Autodesk Fusion 360 part; units mm, degrees
(part 3 of 6)
sketch "mv_std" plane through (-9.843, 0, 81.8196) normal (0, 1, 0) x (1, 0, 0)
  line L0 (174.293, 88.8196) -> (174.293, 74.8196)
  line L1 (40.943, 88.8196) -> (40.943, 74.8196)
  line L2 (131.143, 74.8196) -> (131.143, 88.8196)
  line L3 (112.093, 74.8196) -> (112.093, 88.8196)
  line L4 (35.893, 88.8196) -> (21.893, 88.8196)
  line L5 (98.093, 88.8196) -> (98.093, 74.8196)
  line L6 (2.843, 74.8196) -> (16.843, 74.8196)
  line L7 (174.293, 74.8196) -> (188.293, 74.8196)
  line L8 (2.843, 88.8196) -> (2.843, 74.8196)
  line L9 (21.893, 88.8196) -> (21.893, 74.8196)
  line L10 (150.193, 74.8196) -> (150.193, 88.8196)
  line L11 (16.843, 88.8196) -> (2.843, 88.8196)
  line L12 (59.993, 88.8196) -> (59.993, 74.8196)
  line L13 (131.143, 88.8196) -> (117.143, 88.8196)
  line L14 (98.093, 74.8196) -> (112.093, 74.8196)
  line L15 (21.893, 74.8196) -> (35.893, 74.8196)
  line L16 (35.893, 74.8196) -> (35.893, 88.8196)
  line L17 (188.293, 88.8196) -> (174.293, 88.8196)
  line L18 (59.993, 74.8196) -> (73.993, 74.8196)
  line L19 (188.293, 74.8196) -> (188.293, 88.8196)
  line L20 (16.843, 74.8196) -> (16.843, 88.8196)
  line L21 (54.943, 74.8196) -> (54.943, 88.8196)
  line L22 (73.993, 74.8196) -> (73.993, 88.8196)
  line L23 (73.993, 88.8196) -> (59.993, 88.8196)
  line L24 (40.943, 74.8196) -> (54.943, 74.8196)
  line L25 (117.143, 74.8196) -> (131.143, 74.8196)
  line L26 (54.943, 88.8196) -> (40.943, 88.8196)
  line L27 (155.243, 88.8196) -> (155.243, 74.8196)
  line L28 (136.193, 74.8196) -> (150.193, 74.8196)
  line L29 (112.093, 88.8196) -> (98.093, 88.8196)
  line L30 (79.043, 88.8196) -> (79.043, 74.8196)
  line L31 (150.193, 88.8196) -> (136.193, 88.8196)
  line L32 (93.043, 74.8196) -> (93.043, 88.8196)
  line L33 (169.243, 74.8196) -> (169.243, 88.8196)
  line L34 (93.043, 88.8196) -> (79.043, 88.8196)
  line L35 (193.343, 88.8196) -> (193.343, 74.8196)
  line L36 (40.6555, 55.7696) -> (40.6555, 69.7696)
  line L37 (79.043, 74.8196) -> (93.043, 74.8196)
  line L38 (19.2242, 55.7696) -> (19.2242, 69.7696)
  line L39 (117.143, 88.8196) -> (117.143, 74.8196)
  line L40 (26.6555, 55.7696) -> (40.6555, 55.7696)
  line L41 (26.6555, 69.7696) -> (26.6555, 55.7696)
  line L42 (207.343, 74.8196) -> (207.343, 88.8196)
  line L43 (155.243, 74.8196) -> (169.243, 74.8196)
  line L44 (219.5367, 88.8196) -> (219.5367, 74.8196)
  line L45 (207.343, 88.8196) -> (193.343, 88.8196)
  line L46 (45.7055, 55.7696) -> (59.7055, 55.7696)
  line L47 (233.5367, 88.8196) -> (219.5367, 88.8196)
  line L48 (19.2242, 69.7696) -> (5.2242, 69.7696)
  line L49 (59.7055, 69.7696) -> (45.7055, 69.7696)
  line L50 (59.7055, 55.7696) -> (59.7055, 69.7696)
  line L51 (136.193, 88.8196) -> (136.193, 74.8196)
  line L52 (219.5367, 74.8196) -> (233.5367, 74.8196)
  line L53 (5.2242, 55.7696) -> (19.2242, 55.7696)
  line L54 (5.2242, 69.7696) -> (5.2242, 55.7696)
  line L55 (193.343, 74.8196) -> (207.343, 74.8196)
  line L56 (233.5367, 74.8196) -> (233.5367, 88.8196)
  line L57 (40.6555, 69.7696) -> (26.6555, 69.7696)
  line L58 (169.243, 88.8196) -> (155.243, 88.8196)
  line L59 (160.0055, 69.7696) -> (160.0055, 55.7696)
  line L60 (9.9867, 50.7196) -> (9.9867, 36.7196)
  line L61 (97.8055, 55.7696) -> (97.8055, 69.7696)
  line L62 (78.7555, 55.7696) -> (78.7555, 69.7696)
  line L63 (135.9055, 55.7696) -> (135.9055, 69.7696)
  line L64 (235.918, 69.7696) -> (221.918, 69.7696)
  line L65 (45.7055, 69.7696) -> (45.7055, 55.7696)
  line L66 (36.1805, 36.7196) -> (50.1805, 36.7196)
  line L67 (50.1805, 36.7196) -> (50.1805, 50.7196)
  line L68 (107.3305, 36.7196) -> (107.3305, 50.7196)
  line L69 (140.9555, 55.7696) -> (154.9555, 55.7696)
  line L70 (107.3305, 50.7196) -> (93.3305, 50.7196)
  line L71 (126.3805, 36.7196) -> (126.3805, 50.7196)
  line L72 (36.1805, 50.7196) -> (36.1805, 36.7196)
  line L73 (198.1055, 55.7696) -> (212.1055, 55.7696)
  line L74 (64.7555, 55.7696) -> (78.7555, 55.7696)
  line L75 (78.7555, 69.7696) -> (64.7555, 69.7696)
  line L76 (121.9055, 55.7696) -> (135.9055, 55.7696)
  line L77 (9.9867, 36.7196) -> (23.9867, 36.7196)
  line L78 (145.4305, 36.7196) -> (145.4305, 50.7196)
  line L79 (116.8555, 69.7696) -> (102.8555, 69.7696)
  line L80 (164.4805, 50.7196) -> (150.4805, 50.7196)
  line L81 (112.3805, 36.7196) -> (126.3805, 36.7196)
  line L82 (112.3805, 50.7196) -> (112.3805, 36.7196)
  line L83 (131.4305, 36.7196) -> (145.4305, 36.7196)
  line L84 (93.3305, 50.7196) -> (93.3305, 36.7196)
  line L85 (179.0555, 55.7696) -> (193.0555, 55.7696)
  line L86 (164.4805, 36.7196) -> (164.4805, 50.7196)
  line L87 (102.8555, 69.7696) -> (102.8555, 55.7696)
  line L88 (23.9867, 50.7196) -> (9.9867, 50.7196)
  line L89 (74.2805, 50.7196) -> (74.2805, 36.7196)
  line L90 (121.9055, 69.7696) -> (121.9055, 55.7696)
  line L91 (140.9555, 69.7696) -> (140.9555, 55.7696)
  line L92 (126.3805, 50.7196) -> (112.3805, 50.7196)
  line L93 (145.4305, 50.7196) -> (131.4305, 50.7196)
  line L94 (174.0055, 55.7696) -> (174.0055, 69.7696)
  line L95 (50.1805, 50.7196) -> (36.1805, 50.7196)
  line L96 (150.4805, 50.7196) -> (150.4805, 36.7196)
  line L97 (83.8055, 55.7696) -> (97.8055, 55.7696)
  line L98 (97.8055, 69.7696) -> (83.8055, 69.7696)
  line L99 (83.8055, 69.7696) -> (83.8055, 55.7696)
  line L100 (193.0555, 69.7696) -> (179.0555, 69.7696)
  line L101 (235.918, 55.7696) -> (235.918, 69.7696)
  line L102 (174.0055, 69.7696) -> (160.0055, 69.7696)
  line L103 (64.7555, 69.7696) -> (64.7555, 55.7696)
  line L104 (150.4805, 36.7196) -> (164.4805, 36.7196)
  line L105 (74.2805, 36.7196) -> (88.2805, 36.7196)
  line L106 (212.1055, 69.7696) -> (198.1055, 69.7696)
  line L107 (131.4305, 50.7196) -> (131.4305, 36.7196)
  line L108 (154.9555, 55.7696) -> (154.9555, 69.7696)
  line L109 (179.0555, 69.7696) -> (179.0555, 55.7696)
  line L110 (212.1055, 55.7696) -> (212.1055, 69.7696)
  line L111 (154.9555, 69.7696) -> (140.9555, 69.7696)
  line L112 (116.8555, 55.7696) -> (116.8555, 69.7696)
  line L113 (193.0555, 55.7696) -> (193.0555, 69.7696)
  line L114 (31.418, 17.6696) -> (45.418, 17.6696)
  line L115 (57.6117, 31.6696) -> (57.6117, 17.6696)
  line L116 (169.5305, 50.7196) -> (169.5305, 36.7196)
  line L117 (153.8685, 17.6696) -> (153.8685, 32.6696)
  line L118 (69.2305, 36.7196) -> (69.2305, 50.7196)
  line L119 (233.5367, 31.6696) -> (219.5367, 31.6696)
  line L120 (82.5112, 17.6696) -> (89.5112, 17.6696)
  line L121 (221.918, 69.7696) -> (221.918, 55.7696)
  line L122 (57.6117, 17.6696) -> (71.6117, 17.6696)
  line L123 (131.4305, 17.6696) -> (145.4305, 17.6696)
  line L124 (240.6805, 36.7196) -> (240.6805, 50.7196)
  line L125 (188.5805, 31.6696) -> (188.5805, 17.6696)
  line L126 (145.4305, 31.6696) -> (131.4305, 31.6696)
  line L127 (183.5305, 36.7196) -> (183.5305, 50.7196)
  line L128 (221.918, 55.7696) -> (235.918, 55.7696)
  line L129 (207.6305, 36.7196) -> (221.6305, 36.7196)
  line L130 (19.2242, 31.6696) -> (5.2242, 31.6696)
  line L131 (202.5805, 36.7196) -> (202.5805, 50.7196)
  line L132 (71.6117, 31.6696) -> (57.6117, 31.6696)
  line L133 (219.5367, 17.6696) -> (233.5367, 17.6696)
  line L134 (89.5112, 17.6696) -> (89.5112, 32.6696)
  line L135 (226.6805, 50.7196) -> (226.6805, 36.7196)
  line L136 (55.2305, 50.7196) -> (55.2305, 36.7196)
  line L137 (93.3305, 36.7196) -> (107.3305, 36.7196)
  line L138 (122.9925, 17.6696) -> (129.9925, 17.6696)
  line L139 (198.1055, 69.7696) -> (198.1055, 55.7696)
  line L140 (135.9055, 69.7696) -> (121.9055, 69.7696)
  line L141 (113.3872, 32.6696) -> (106.3872, 32.6696)
  line L142 (129.9925, 17.6696) -> (129.9925, 32.6696)
  line L143 (207.6305, 50.7196) -> (207.6305, 36.7196)
  line L144 (5.2242, 31.6696) -> (5.2242, 17.6696)
  line L145 (188.5805, 50.7196) -> (188.5805, 36.7196)
  line L146 (90.9492, 17.6696) -> (104.9492, 17.6696)
  line L147 (162.3867, 17.6696) -> (176.3867, 17.6696)
  line L148 (202.5805, 50.7196) -> (188.5805, 50.7196)
  line L149 (162.3867, 31.6696) -> (162.3867, 17.6696)
  line L150 (183.5305, 50.7196) -> (169.5305, 50.7196)
  line L151 (19.2242, 17.6696) -> (19.2242, 31.6696)
  line L152 (90.9492, 31.6696) -> (90.9492, 17.6696)
  line L153 (176.3867, 17.6696) -> (176.3867, 31.6696)
  line L154 (82.5112, 32.6696) -> (82.5112, 17.6696)
  line L155 (88.2805, 36.7196) -> (88.2805, 50.7196)
  line L156 (160.0055, 55.7696) -> (174.0055, 55.7696)
  line L157 (221.6305, 36.7196) -> (221.6305, 50.7196)
  line L158 (129.9925, 32.6696) -> (122.9925, 32.6696)
  line L159 (71.6117, 17.6696) -> (71.6117, 31.6696)
  line L160 (233.5367, 17.6696) -> (233.5367, 31.6696)
  line L161 (102.8555, 55.7696) -> (116.8555, 55.7696)
  line L162 (188.5805, 36.7196) -> (202.5805, 36.7196)
  line L163 (202.5805, 17.6696) -> (202.5805, 31.6696)
  line L164 (113.3872, 17.6696) -> (113.3872, 32.6696)
  line L165 (219.5367, 31.6696) -> (219.5367, 17.6696)
  line L166 (45.418, 17.6696) -> (45.418, 31.6696)
  line L167 (55.2305, 36.7196) -> (69.2305, 36.7196)
  line L168 (88.2805, 50.7196) -> (74.2805, 50.7196)
  line L169 (176.3867, 31.6696) -> (162.3867, 31.6696)
  line L170 (146.8685, 32.6696) -> (146.8685, 17.6696)
  line L171 (23.9867, 36.7196) -> (23.9867, 50.7196)
  line L172 (240.6805, 50.7196) -> (226.6805, 50.7196)
  line L173 (221.6305, 50.7196) -> (207.6305, 50.7196)
  line L174 (106.3872, 32.6696) -> (106.3872, 17.6696)
  line L175 (226.6805, 36.7196) -> (240.6805, 36.7196)
  line L176 (45.418, 31.6696) -> (31.418, 31.6696)
  line L177 (69.2305, 50.7196) -> (55.2305, 50.7196)
  line L178 (169.5305, 36.7196) -> (183.5305, 36.7196)
  line L179 (106.3872, 17.6696) -> (113.3872, 17.6696)
  line L180 (188.5805, 17.6696) -> (202.5805, 17.6696)
  line L181 (31.418, 31.6696) -> (31.418, 17.6696)
  line L182 (104.9492, 17.6696) -> (104.9492, 31.6696)
  line L183 (202.5805, 31.6696) -> (188.5805, 31.6696)
  line L184 (104.9492, 31.6696) -> (90.9492, 31.6696)
  line L185 (89.5112, 32.6696) -> (82.5112, 32.6696)
  line L186 (5.2242, 17.6696) -> (19.2242, 17.6696)
  line L187 (122.9925, 32.6696) -> (122.9925, 17.6696)
  line L188 (146.8685, 17.6696) -> (153.8685, 17.6696)
  line L189 (153.8685, 32.6696) -> (146.8685, 32.6696)
  line L190 (131.4305, 31.6696) -> (131.4305, 17.6696)
  line L191 (145.4305, 17.6696) -> (145.4305, 31.6696)
  point P0 (9.843, 81.8196)
sketch "mv_southpaw" plane through (-7.7091, 0, 89.8505) normal (0, 1, 0) x (1, 0, 0)
  line L0 (186.1591, 82.8505) -> (186.1591, 96.8505)
  line L1 (109.9591, 96.8505) -> (95.9591, 96.8505)
  line L2 (14.7091, 82.8505) -> (14.7091, 96.8505)
  line L3 (19.7591, 96.8505) -> (19.7591, 82.8505)
  line L4 (38.8091, 96.8505) -> (38.8091, 82.8505)
  line L5 (33.7591, 82.8505) -> (33.7591, 96.8505)
  line L6 (129.0091, 96.8505) -> (115.0091, 96.8505)
  line L7 (205.2091, 96.8505) -> (191.2091, 96.8505)
  line L8 (172.1591, 82.8505) -> (186.1591, 82.8505)
  line L9 (167.1091, 82.8505) -> (167.1091, 96.8505)
  line L10 (109.9591, 82.8505) -> (109.9591, 96.8505)
  line L11 (134.0591, 96.8505) -> (134.0591, 82.8505)
  line L12 (57.8591, 82.8505) -> (71.8591, 82.8505)
  line L13 (57.8591, 96.8505) -> (57.8591, 82.8505)
  line L14 (19.7591, 82.8505) -> (33.7591, 82.8505)
  line L15 (38.8091, 82.8505) -> (52.8091, 82.8505)
  line L16 (172.1591, 96.8505) -> (172.1591, 82.8505)
  line L17 (71.8591, 96.8505) -> (57.8591, 96.8505)
  line L18 (129.0091, 82.8505) -> (129.0091, 96.8505)
  line L19 (76.9091, 96.8505) -> (76.9091, 82.8505)
  line L20 (115.0091, 82.8505) -> (129.0091, 82.8505)
  line L21 (33.7591, 96.8505) -> (19.7591, 96.8505)
  line L22 (186.1591, 96.8505) -> (172.1591, 96.8505)
  line L23 (90.9091, 82.8505) -> (90.9091, 96.8505)
  line L24 (167.1091, 96.8505) -> (153.1091, 96.8505)
  line L25 (148.0591, 96.8505) -> (134.0591, 96.8505)
  line L26 (148.0591, 82.8505) -> (148.0591, 96.8505)
  line L27 (191.2091, 82.8505) -> (205.2091, 82.8505)
  line L28 (134.0591, 82.8505) -> (148.0591, 82.8505)
  line L29 (95.9591, 96.8505) -> (95.9591, 82.8505)
  line L30 (95.9591, 82.8505) -> (109.9591, 82.8505)
  line L31 (90.9091, 96.8505) -> (76.9091, 96.8505)
  line L32 (14.7091, 96.8505) -> (0.7091, 96.8505)
  line L33 (0.7091, 96.8505) -> (0.7091, 82.8505)
  line L34 (153.1091, 82.8505) -> (167.1091, 82.8505)
  line L35 (0.7091, 82.8505) -> (14.7091, 82.8505)
  line L36 (153.1091, 96.8505) -> (153.1091, 82.8505)
  line L37 (52.8091, 82.8505) -> (52.8091, 96.8505)
  line L38 (115.0091, 96.8505) -> (115.0091, 82.8505)
  line L39 (52.8091, 96.8505) -> (38.8091, 96.8505)
  line L40 (71.8591, 82.8505) -> (71.8591, 96.8505)
  line L41 (76.9091, 82.8505) -> (90.9091, 82.8505)
  line L42 (205.2091, 82.8505) -> (205.2091, 96.8505)
  line L43 (231.4028, 82.8505) -> (231.4028, 96.8505)
  line L44 (191.2091, 96.8505) -> (191.2091, 82.8505)
  line L45 (231.4028, 96.8505) -> (217.4028, 96.8505)
  line L46 (217.4028, 82.8505) -> (231.4028, 82.8505)
  line L47 (217.4028, 96.8505) -> (217.4028, 82.8505)
  line L48 (3.0903, 63.8005) -> (17.0903, 63.8005)
  line L49 (17.0903, 63.8005) -> (17.0903, 77.8005)
  line L50 (24.5216, 63.8005) -> (38.5216, 63.8005)
  line L51 (17.0903, 77.8005) -> (3.0903, 77.8005)
  line L52 (24.5216, 77.8005) -> (24.5216, 63.8005)
  line L53 (43.5716, 63.8005) -> (57.5716, 63.8005)
  line L54 (3.0903, 77.8005) -> (3.0903, 63.8005)
  line L55 (57.5716, 77.8005) -> (43.5716, 77.8005)
  line L56 (38.5216, 77.8005) -> (24.5216, 77.8005)
  line L57 (38.5216, 63.8005) -> (38.5216, 77.8005)
  line L58 (157.8716, 63.8005) -> (171.8716, 63.8005)
  line L59 (124.2466, 58.7505) -> (110.2466, 58.7505)
  line L60 (152.8216, 77.8005) -> (138.8216, 77.8005)
  line L61 (48.0466, 58.7505) -> (34.0466, 58.7505)
  line L62 (219.7841, 77.8005) -> (219.7841, 63.8005)
  line L63 (7.8528, 44.7505) -> (21.8528, 44.7505)
  line L64 (133.7716, 77.8005) -> (119.7716, 77.8005)
  line L65 (21.8528, 44.7505) -> (21.8528, 58.7505)
  line L66 (209.9716, 77.8005) -> (195.9716, 77.8005)
  line L67 (34.0466, 58.7505) -> (34.0466, 44.7505)
  line L68 (53.0966, 58.7505) -> (53.0966, 44.7505)
  line L69 (162.3466, 44.7505) -> (162.3466, 58.7505)
  line L70 (119.7716, 63.8005) -> (133.7716, 63.8005)
  line L71 (114.7216, 77.8005) -> (100.7216, 77.8005)
  line L72 (48.0466, 44.7505) -> (48.0466, 58.7505)
  line L73 (43.5716, 77.8005) -> (43.5716, 63.8005)
  line L74 (129.2966, 58.7505) -> (129.2966, 44.7505)
  line L75 (157.8716, 77.8005) -> (157.8716, 63.8005)
  line L76 (76.6216, 63.8005) -> (76.6216, 77.8005)
  line L77 (86.1466, 44.7505) -> (86.1466, 58.7505)
  line L78 (176.9216, 63.8005) -> (190.9216, 63.8005)
  line L79 (171.8716, 63.8005) -> (171.8716, 77.8005)
  line L80 (62.6216, 63.8005) -> (76.6216, 63.8005)
  line L81 (62.6216, 77.8005) -> (62.6216, 63.8005)
  line L82 (110.2466, 44.7505) -> (124.2466, 44.7505)
  line L83 (57.5716, 63.8005) -> (57.5716, 77.8005)
  line L84 (21.8528, 58.7505) -> (7.8528, 58.7505)
  line L85 (100.7216, 77.8005) -> (100.7216, 63.8005)
  line L86 (76.6216, 77.8005) -> (62.6216, 77.8005)
  line L87 (7.8528, 58.7505) -> (7.8528, 44.7505)
  line L88 (86.1466, 58.7505) -> (72.1466, 58.7505)
  line L89 (124.2466, 44.7505) -> (124.2466, 58.7505)
  line L90 (143.2966, 44.7505) -> (143.2966, 58.7505)
  line L91 (162.3466, 58.7505) -> (148.3466, 58.7505)
  line L92 (119.7716, 77.8005) -> (119.7716, 63.8005)
  line L93 (152.8216, 63.8005) -> (152.8216, 77.8005)
  line L94 (110.2466, 58.7505) -> (110.2466, 44.7505)
  line L95 (138.8216, 77.8005) -> (138.8216, 63.8005)
  line L96 (190.9216, 63.8005) -> (190.9216, 77.8005)
  line L97 (72.1466, 44.7505) -> (86.1466, 44.7505)
  line L98 (190.9216, 77.8005) -> (176.9216, 77.8005)
  line L99 (143.2966, 58.7505) -> (129.2966, 58.7505)
  line L100 (133.7716, 63.8005) -> (133.7716, 77.8005)
  line L101 (67.0966, 44.7505) -> (67.0966, 58.7505)
  line L102 (171.8716, 77.8005) -> (157.8716, 77.8005)
  line L103 (91.1966, 58.7505) -> (91.1966, 44.7505)
  line L104 (176.9216, 77.8005) -> (176.9216, 63.8005)
  line L105 (72.1466, 58.7505) -> (72.1466, 44.7505)
  line L106 (100.7216, 63.8005) -> (114.7216, 63.8005)
  line L107 (34.0466, 44.7505) -> (48.0466, 44.7505)
  line L108 (81.6716, 77.8005) -> (81.6716, 63.8005)
  line L109 (233.7841, 77.8005) -> (219.7841, 77.8005)
  line L110 (105.1966, 44.7505) -> (105.1966, 58.7505)
  line L111 (91.1966, 44.7505) -> (105.1966, 44.7505)
  line L112 (81.6716, 63.8005) -> (95.6716, 63.8005)
  line L113 (129.2966, 44.7505) -> (143.2966, 44.7505)
  line L114 (148.3466, 44.7505) -> (162.3466, 44.7505)
  line L115 (95.6716, 77.8005) -> (81.6716, 77.8005)
  line L116 (105.1966, 58.7505) -> (91.1966, 58.7505)
  line L117 (209.9716, 63.8005) -> (209.9716, 77.8005)
  line L118 (67.0966, 58.7505) -> (53.0966, 58.7505)
  line L119 (195.9716, 77.8005) -> (195.9716, 63.8005)
  line L120 (80.3773, 40.7005) -> (80.3773, 25.7005)
  line L121 (200.4466, 39.7005) -> (186.4466, 39.7005)
  line L122 (205.4966, 44.7505) -> (219.4966, 44.7505)
  line L123 (114.7216, 63.8005) -> (114.7216, 77.8005)
  line L124 (238.5466, 58.7505) -> (224.5466, 58.7505)
  line L125 (38.8091, 39.7005) -> (38.8091, 25.7005)
  line L126 (104.2533, 25.7005) -> (111.2533, 25.7005)
  line L127 (87.3773, 40.7005) -> (80.3773, 40.7005)
  line L128 (143.2966, 39.7005) -> (129.2966, 39.7005)
  line L129 (200.4466, 44.7505) -> (200.4466, 58.7505)
  line L130 (144.7346, 25.7005) -> (151.7346, 25.7005)
  line L131 (205.4966, 58.7505) -> (205.4966, 44.7505)
  line L132 (33.7591, 25.7005) -> (33.7591, 39.7005)
  line L133 (0.7091, 39.7005) -> (0.7091, 25.7005)
  line L134 (88.8153, 39.7005) -> (88.8153, 25.7005)
  line L135 (38.8091, 25.7005) -> (52.8091, 25.7005)
  line L136 (111.2533, 25.7005) -> (111.2533, 40.7005)
  line L137 (233.7841, 63.8005) -> (233.7841, 77.8005)
  line L138 (160.2528, 39.7005) -> (160.2528, 25.7005)
  line L139 (144.7346, 40.7005) -> (144.7346, 25.7005)
  line L140 (138.8216, 63.8005) -> (152.8216, 63.8005)
  line L141 (186.4466, 58.7505) -> (186.4466, 44.7505)
  line L142 (219.7841, 63.8005) -> (233.7841, 63.8005)
  line L143 (53.0966, 44.7505) -> (67.0966, 44.7505)
  line L144 (120.8586, 40.7005) -> (120.8586, 25.7005)
  line L145 (174.2528, 39.7005) -> (160.2528, 39.7005)
  line L146 (129.2966, 25.7005) -> (143.2966, 25.7005)
  line L147 (33.7591, 39.7005) -> (19.7591, 39.7005)
  line L148 (174.2528, 25.7005) -> (174.2528, 39.7005)
  line L149 (151.7346, 25.7005) -> (151.7346, 40.7005)
  line L150 (186.4466, 25.7005) -> (200.4466, 25.7005)
  line L151 (87.3773, 25.7005) -> (87.3773, 40.7005)
  line L152 (88.8153, 25.7005) -> (102.8153, 25.7005)
  line L153 (200.4466, 25.7005) -> (200.4466, 39.7005)
  line L154 (186.4466, 44.7505) -> (200.4466, 44.7505)
  line L155 (151.7346, 40.7005) -> (144.7346, 40.7005)
  line L156 (127.8586, 40.7005) -> (120.8586, 40.7005)
  line L157 (95.6716, 63.8005) -> (95.6716, 77.8005)
  line L158 (127.8586, 25.7005) -> (127.8586, 40.7005)
  line L159 (195.9716, 63.8005) -> (209.9716, 63.8005)
  line L160 (57.8591, 39.7005) -> (57.8591, 25.7005)
  line L161 (181.3966, 44.7505) -> (181.3966, 58.7505)
  line L162 (57.8591, 25.7005) -> (71.8591, 25.7005)
  line L163 (80.3773, 25.7005) -> (87.3773, 25.7005)
  line L164 (0.7091, 25.7005) -> (14.7091, 25.7005)
  line L165 (102.8153, 39.7005) -> (88.8153, 39.7005)
  line L166 (71.8591, 25.7005) -> (71.8591, 39.7005)
  line L167 (167.3966, 58.7505) -> (167.3966, 44.7505)
  line L168 (19.7591, 25.7005) -> (33.7591, 25.7005)
  line L169 (52.8091, 25.7005) -> (52.8091, 39.7005)
  line L170 (148.3466, 58.7505) -> (148.3466, 44.7505)
  line L171 (224.5466, 58.7505) -> (224.5466, 44.7505)
  line L172 (52.8091, 39.7005) -> (38.8091, 39.7005)
  line L173 (129.2966, 39.7005) -> (129.2966, 25.7005)
  line L174 (104.2533, 40.7005) -> (104.2533, 25.7005)
  line L175 (231.4028, 39.7005) -> (217.4028, 39.7005)
  line L176 (14.7091, 25.7005) -> (14.7091, 39.7005)
  line L177 (143.2966, 25.7005) -> (143.2966, 39.7005)
  line L178 (167.3966, 44.7505) -> (181.3966, 44.7505)
  line L179 (219.4966, 58.7505) -> (205.4966, 58.7505)
  line L180 (71.8591, 39.7005) -> (57.8591, 39.7005)
  line L181 (200.4466, 58.7505) -> (186.4466, 58.7505)
  line L182 (217.4028, 39.7005) -> (217.4028, 25.7005)
  line L183 (238.5466, 44.7505) -> (238.5466, 58.7505)
  line L184 (231.4028, 25.7005) -> (231.4028, 39.7005)
  line L185 (224.5466, 44.7505) -> (238.5466, 44.7505)
  line L186 (120.8586, 25.7005) -> (127.8586, 25.7005)
  line L187 (160.2528, 25.7005) -> (174.2528, 25.7005)
  line L188 (181.3966, 58.7505) -> (167.3966, 58.7505)
  line L189 (19.7591, 39.7005) -> (19.7591, 25.7005)
  line L190 (217.4028, 25.7005) -> (231.4028, 25.7005)
  line L191 (111.2533, 40.7005) -> (104.2533, 40.7005)
  line L192 (102.8153, 25.7005) -> (102.8153, 39.7005)
  line L193 (186.4466, 39.7005) -> (186.4466, 25.7005)
  line L194 (14.7091, 39.7005) -> (0.7091, 39.7005)
  line L195 (219.4966, 44.7505) -> (219.4966, 58.7505)
  point P0 (7.7091, 89.8505)
sketch "mv_arrows" plane through (-8.3913, 0, 73.9082) normal (0, 1, 0) x (1, 0, 0)
  line L0 (91.5913, 80.9082) -> (77.5913, 80.9082)
  line L1 (115.6913, 80.9082) -> (115.6913, 66.9082)
  line L2 (77.5913, 80.9082) -> (77.5913, 66.9082)
  line L3 (58.5413, 66.9082) -> (72.5413, 66.9082)
  line L4 (134.7413, 80.9082) -> (134.7413, 66.9082)
  line L5 (72.5413, 66.9082) -> (72.5413, 80.9082)
  line L6 (72.5413, 80.9082) -> (58.5413, 80.9082)
  line L7 (96.6413, 66.9082) -> (110.6413, 66.9082)
  line L8 (91.5913, 66.9082) -> (91.5913, 80.9082)
  line L9 (172.8413, 66.9082) -> (186.8413, 66.9082)
  line L10 (77.5913, 66.9082) -> (91.5913, 66.9082)
  line L11 (34.4413, 66.9082) -> (34.4413, 80.9082)
  line L12 (110.6413, 80.9082) -> (96.6413, 80.9082)
  line L13 (20.4413, 66.9082) -> (34.4413, 66.9082)
  line L14 (186.8413, 80.9082) -> (172.8413, 80.9082)
  line L15 (34.4413, 80.9082) -> (20.4413, 80.9082)
  line L16 (53.4913, 80.9082) -> (39.4913, 80.9082)
  line L17 (186.8413, 66.9082) -> (186.8413, 80.9082)
  line L18 (39.4913, 66.9082) -> (53.4913, 66.9082)
  line L19 (129.6913, 66.9082) -> (129.6913, 80.9082)
  line L20 (153.7913, 80.9082) -> (153.7913, 66.9082)
  line L21 (115.6913, 66.9082) -> (129.6913, 66.9082)
  line L22 (1.3913, 66.9082) -> (15.3913, 66.9082)
  line L23 (205.8913, 66.9082) -> (205.8913, 80.9082)
  line L24 (172.8413, 80.9082) -> (172.8413, 66.9082)
  line L25 (110.6413, 66.9082) -> (110.6413, 80.9082)
  line L26 (96.6413, 80.9082) -> (96.6413, 66.9082)
  line L27 (129.6913, 80.9082) -> (115.6913, 80.9082)
  line L28 (39.4913, 80.9082) -> (39.4913, 66.9082)
  line L29 (167.7913, 80.9082) -> (153.7913, 80.9082)
  line L30 (20.4413, 80.9082) -> (20.4413, 66.9082)
  line L31 (134.7413, 66.9082) -> (148.7413, 66.9082)
  line L32 (191.8913, 66.9082) -> (205.8913, 66.9082)
  line L33 (191.8913, 80.9082) -> (191.8913, 66.9082)
  line L34 (58.5413, 80.9082) -> (58.5413, 66.9082)
  line L35 (232.0851, 80.9082) -> (218.0851, 80.9082)
  line L36 (232.0851, 66.9082) -> (232.0851, 80.9082)
  line L37 (15.3913, 80.9082) -> (1.3913, 80.9082)
  line L38 (218.0851, 66.9082) -> (232.0851, 66.9082)
  line L39 (15.3913, 66.9082) -> (15.3913, 80.9082)
  line L40 (167.7913, 66.9082) -> (167.7913, 80.9082)
  line L41 (3.7726, 47.8582) -> (17.7726, 47.8582)
  line L42 (153.7913, 66.9082) -> (167.7913, 66.9082)
  line L43 (148.7413, 66.9082) -> (148.7413, 80.9082)
  line L44 (218.0851, 80.9082) -> (218.0851, 66.9082)
  line L45 (17.7726, 61.8582) -> (3.7726, 61.8582)
  line L46 (148.7413, 80.9082) -> (134.7413, 80.9082)
  line L47 (53.4913, 66.9082) -> (53.4913, 80.9082)
  line L48 (1.3913, 80.9082) -> (1.3913, 66.9082)
  line L49 (3.7726, 61.8582) -> (3.7726, 47.8582)
  line L50 (205.8913, 80.9082) -> (191.8913, 80.9082)
  line L51 (105.8788, 42.8082) -> (91.8788, 42.8082)
  line L52 (115.4038, 47.8582) -> (115.4038, 61.8582)
  line L53 (77.3038, 61.8582) -> (63.3038, 61.8582)
  line L54 (182.0788, 42.8082) -> (168.0788, 42.8082)
  line L55 (39.2038, 47.8582) -> (39.2038, 61.8582)
  line L56 (101.4038, 47.8582) -> (115.4038, 47.8582)
  line L57 (63.3038, 47.8582) -> (77.3038, 47.8582)
  line L58 (77.3038, 47.8582) -> (77.3038, 61.8582)
  line L59 (120.4538, 47.8582) -> (134.4538, 47.8582)
  line L60 (120.4538, 61.8582) -> (120.4538, 47.8582)
  line L61 (44.2538, 47.8582) -> (58.2538, 47.8582)
  line L62 (82.3538, 61.8582) -> (82.3538, 47.8582)
  line L63 (63.3038, 61.8582) -> (63.3038, 47.8582)
  line L64 (101.4038, 61.8582) -> (101.4038, 47.8582)
  line L65 (25.2038, 61.8582) -> (25.2038, 47.8582)
  line L66 (39.2038, 61.8582) -> (25.2038, 61.8582)
  line L67 (153.5038, 61.8582) -> (139.5038, 61.8582)
  line L68 (58.2538, 61.8582) -> (44.2538, 61.8582)
  line L69 (153.5038, 47.8582) -> (153.5038, 61.8582)
  line L70 (115.4038, 61.8582) -> (101.4038, 61.8582)
  line L71 (17.7726, 9.7582) -> (17.7726, 23.7582)
  line L72 (53.7788, 42.8082) -> (53.7788, 28.8082)
  line L73 (158.5538, 61.8582) -> (158.5538, 47.8582)
  line L74 (129.9788, 42.8082) -> (129.9788, 28.8082)
  line L75 (134.4538, 61.8582) -> (120.4538, 61.8582)
  line L76 (34.7288, 42.8082) -> (34.7288, 28.8082)
  line L77 (72.8288, 42.8082) -> (72.8288, 28.8082)
  line L78 (44.2538, 61.8582) -> (44.2538, 47.8582)
  line L79 (58.2538, 47.8582) -> (58.2538, 61.8582)
  line L80 (191.6038, 47.8582) -> (191.6038, 61.8582)
  line L81 (172.5538, 61.8582) -> (158.5538, 61.8582)
  line L82 (91.8788, 42.8082) -> (91.8788, 28.8082)
  line L83 (96.3538, 61.8582) -> (82.3538, 61.8582)
  line L84 (67.7788, 42.8082) -> (53.7788, 42.8082)
  line L85 (172.5538, 47.8582) -> (172.5538, 61.8582)
  line L86 (187.1288, 28.8082) -> (201.1288, 28.8082)
  line L87 (82.3538, 47.8582) -> (96.3538, 47.8582)
  line L88 (163.0288, 42.8082) -> (149.0288, 42.8082)
  line L89 (191.6038, 61.8582) -> (177.6038, 61.8582)
  line L90 (177.6038, 61.8582) -> (177.6038, 47.8582)
  line L91 (22.5351, 42.8082) -> (8.5351, 42.8082)
  line L92 (158.5538, 47.8582) -> (172.5538, 47.8582)
  line L93 (96.3538, 47.8582) -> (96.3538, 61.8582)
  line L94 (206.1788, 28.8082) -> (220.1788, 28.8082)
  line L95 (139.5038, 47.8582) -> (153.5038, 47.8582)
  line L96 (182.0788, 28.8082) -> (182.0788, 42.8082)
  line L97 (86.8288, 28.8082) -> (86.8288, 42.8082)
  line L98 (67.7788, 28.8082) -> (67.7788, 42.8082)
  line L99 (134.4538, 47.8582) -> (134.4538, 61.8582)
  line L100 (17.7726, 47.8582) -> (17.7726, 61.8582)
  line L101 (25.2038, 47.8582) -> (39.2038, 47.8582)
  line L102 (139.5038, 61.8582) -> (139.5038, 47.8582)
  line L103 (177.6038, 47.8582) -> (191.6038, 47.8582)
  line L104 (22.5351, 28.8082) -> (22.5351, 42.8082)
  line L105 (89.4976, 9.7582) -> (103.4976, 9.7582)
  line L106 (187.1288, 23.7582) -> (187.1288, 9.7582)
  line L107 (111.9356, 24.7582) -> (104.9356, 24.7582)
  line L108 (48.7288, 42.8082) -> (34.7288, 42.8082)
  line L109 (143.9788, 28.8082) -> (143.9788, 42.8082)
  line L110 (72.8288, 28.8082) -> (86.8288, 28.8082)
  line L111 (152.4168, 24.7582) -> (145.4168, 24.7582)
  line L112 (168.0788, 42.8082) -> (168.0788, 28.8082)
  line L113 (81.0596, 9.7582) -> (88.0596, 9.7582)
  line L114 (124.9288, 28.8082) -> (124.9288, 42.8082)
  line L115 (8.5351, 28.8082) -> (22.5351, 28.8082)
  line L116 (149.0288, 42.8082) -> (149.0288, 28.8082)
  line L117 (163.0288, 28.8082) -> (163.0288, 42.8082)
  line L118 (143.9788, 42.8082) -> (129.9788, 42.8082)
  line L119 (225.2288, 42.8082) -> (225.2288, 28.8082)
  line L120 (3.7726, 9.7582) -> (17.7726, 9.7582)
  line L121 (168.0788, 28.8082) -> (182.0788, 28.8082)
  line L122 (149.0288, 28.8082) -> (163.0288, 28.8082)
  line L123 (3.7726, 23.7582) -> (3.7726, 9.7582)
  line L124 (129.9788, 28.8082) -> (143.9788, 28.8082)
  line L125 (201.1288, 23.7582) -> (187.1288, 23.7582)
  line L126 (88.0596, 24.7582) -> (81.0596, 24.7582)
  line L127 (225.2288, 23.7582) -> (225.2288, 9.7582)
  line L128 (43.9663, 23.7582) -> (29.9663, 23.7582)
  line L129 (91.8788, 28.8082) -> (105.8788, 28.8082)
  line L130 (105.8788, 28.8082) -> (105.8788, 42.8082)
  line L131 (220.4663, 47.8582) -> (234.4663, 47.8582)
  line L132 (111.9356, 9.7582) -> (111.9356, 24.7582)
  line L133 (163.3163, 23.7582) -> (163.3163, 9.7582)
  line L134 (220.1788, 23.7582) -> (206.1788, 23.7582)
  line L135 (220.4663, 61.8582) -> (220.4663, 47.8582)
  line L136 (43.9663, 9.7582) -> (43.9663, 23.7582)
  line L137 (124.9288, 42.8082) -> (110.9288, 42.8082)
  line L138 (234.4663, 61.8582) -> (220.4663, 61.8582)
  line L139 (187.1288, 42.8082) -> (187.1288, 28.8082)
  line L140 (86.8288, 42.8082) -> (72.8288, 42.8082)
  line L141 (220.1788, 28.8082) -> (220.1788, 42.8082)
  line L142 (48.7288, 28.8082) -> (48.7288, 42.8082)
  line L143 (206.1788, 42.8082) -> (206.1788, 28.8082)
  line L144 (239.2288, 42.8082) -> (225.2288, 42.8082)
  line L145 (53.7788, 28.8082) -> (67.7788, 28.8082)
  line L146 (234.4663, 47.8582) -> (234.4663, 61.8582)
  line L147 (34.7288, 28.8082) -> (48.7288, 28.8082)
  line L148 (8.5351, 42.8082) -> (8.5351, 28.8082)
  line L149 (29.9663, 23.7582) -> (29.9663, 9.7582)
  line L150 (29.9663, 9.7582) -> (43.9663, 9.7582)
  line L151 (196.6538, 47.8582) -> (210.6538, 47.8582)
  line L152 (201.1288, 42.8082) -> (187.1288, 42.8082)
  line L153 (210.6538, 61.8582) -> (196.6538, 61.8582)
  line L154 (110.9288, 28.8082) -> (124.9288, 28.8082)
  line L155 (110.9288, 42.8082) -> (110.9288, 28.8082)
  line L156 (239.2288, 28.8082) -> (239.2288, 42.8082)
  line L157 (201.1288, 28.8082) -> (201.1288, 42.8082)
  line L158 (220.1788, 42.8082) -> (206.1788, 42.8082)
  line L159 (17.7726, 23.7582) -> (3.7726, 23.7582)
  line L160 (210.6538, 47.8582) -> (210.6538, 61.8582)
  line L161 (225.2288, 28.8082) -> (239.2288, 28.8082)
  line L162 (196.6538, 61.8582) -> (196.6538, 47.8582)
  line L163 (145.4168, 9.7582) -> (152.4168, 9.7582)
  line L164 (220.1788, 9.7582) -> (220.1788, 23.7582)
  line L165 (70.1601, 9.7582) -> (70.1601, 23.7582)
  line L166 (103.4976, 9.7582) -> (103.4976, 23.7582)
  line L167 (201.1288, 9.7582) -> (201.1288, 23.7582)
  line L168 (81.0596, 24.7582) -> (81.0596, 9.7582)
  line L169 (145.4168, 24.7582) -> (145.4168, 9.7582)
  line L170 (225.2288, 9.7582) -> (239.2288, 9.7582)
  line L171 (206.1788, 9.7582) -> (220.1788, 9.7582)
  line L172 (239.2288, 23.7582) -> (225.2288, 23.7582)
  line L173 (121.5408, 24.7582) -> (121.5408, 9.7582)
  line L174 (177.3163, 9.7582) -> (177.3163, 23.7582)
  line L175 (103.4976, 23.7582) -> (89.4976, 23.7582)
  line L176 (89.4976, 23.7582) -> (89.4976, 9.7582)
  line L177 (70.1601, 23.7582) -> (56.1601, 23.7582)
  line L178 (163.3163, 9.7582) -> (177.3163, 9.7582)
  line L179 (129.9788, 23.7582) -> (129.9788, 9.7582)
  line L180 (143.9788, 9.7582) -> (143.9788, 23.7582)
  line L181 (104.9356, 24.7582) -> (104.9356, 9.7582)
  line L182 (104.9356, 9.7582) -> (111.9356, 9.7582)
  line L183 (143.9788, 23.7582) -> (129.9788, 23.7582)
  line L184 (152.4168, 9.7582) -> (152.4168, 24.7582)
  line L185 (187.1288, 9.7582) -> (201.1288, 9.7582)
  line L186 (206.1788, 23.7582) -> (206.1788, 9.7582)
  line L187 (56.1601, 9.7582) -> (70.1601, 9.7582)
  line L188 (128.5408, 9.7582) -> (128.5408, 24.7582)
  line L189 (177.3163, 23.7582) -> (163.3163, 23.7582)
  line L190 (56.1601, 23.7582) -> (56.1601, 9.7582)
  line L191 (129.9788, 9.7582) -> (143.9788, 9.7582)
  line L192 (88.0596, 9.7582) -> (88.0596, 24.7582)
  line L193 (239.2288, 9.7582) -> (239.2288, 23.7582)
  line L194 (128.5408, 24.7582) -> (121.5408, 24.7582)
  line L195 (121.5408, 9.7582) -> (128.5408, 9.7582)
  point P0 (8.3913, 73.9082)
sketch "mv_southpaw_arrows" plane through (0, 0, 0) normal (0, 1, 0) x (1, 0, 0)
  line L0 (102.25, 7) -> (88.25, 7)
  line L1 (26.05, 7) -> (12.05, 7)
  line L2 (88.25, 7) -> (88.25, -7)
  line L3 (7, -7) -> (7, 7)
  line L4 (126.35, -7) -> (140.35, -7)
  line L5 (126.35, 7) -> (126.35, -7)
  line L6 (102.25, -7) -> (102.25, 7)
  line L7 (45.1, -7) -> (45.1, 7)
  line L8 (178.45, 7) -> (164.45, 7)
  line L9 (12.05, -7) -> (26.05, -7)
  line L10 (83.2, -7) -> (83.2, 7)
  line L11 (64.15, 7) -> (50.15, 7)
  line L12 (26.05, -7) -> (26.05, 7)
  line L13 (-7, 7) -> (-7, -7)
  line L14 (50.15, -7) -> (64.15, -7)
  line L15 (31.1, -7) -> (45.1, -7)
  line L16 (31.1, 7) -> (31.1, -7)
  line L17 (121.3, -7) -> (121.3, 7)
  line L18 (-7, -7) -> (7, -7)
  line L19 (145.4, 7) -> (145.4, -7)
  line L20 (145.4, -7) -> (159.4, -7)
  line L21 (159.4, 7) -> (145.4, 7)
  line L22 (69.2, 7) -> (69.2, -7)
  line L23 (121.3, 7) -> (107.3, 7)
  line L24 (107.3, -7) -> (121.3, -7)
  line L25 (178.45, -7) -> (178.45, 7)
  line L26 (164.45, 7) -> (164.45, -7)
  line L27 (164.45, -7) -> (178.45, -7)
  line L28 (183.5, -7) -> (197.5, -7)
  line L29 (50.15, 7) -> (50.15, -7)
  line L30 (7, 7) -> (-7, 7)
  line L31 (88.25, -7) -> (102.25, -7)
  line L32 (12.05, 7) -> (12.05, -7)
  line L33 (140.35, 7) -> (126.35, 7)
  line L34 (83.2, 7) -> (69.2, 7)
  line L35 (107.3, 7) -> (107.3, -7)
  line L36 (64.15, -7) -> (64.15, 7)
  line L37 (197.5, 7) -> (183.5, 7)
  line L38 (69.2, -7) -> (83.2, -7)
  line L39 (145.1125, -12.05) -> (131.1125, -12.05)
  line L40 (93.0125, -26.05) -> (107.0125, -26.05)
  line L41 (202.2625, -12.05) -> (188.2625, -12.05)
  line L42 (131.1125, -12.05) -> (131.1125, -26.05)
  line L43 (54.9125, -26.05) -> (68.9125, -26.05)
  line L44 (226.075, -26.05) -> (226.075, -12.05)
  line L45 (164.1625, -26.05) -> (164.1625, -12.05)
  line L46 (0.1438, -45.1) -> (14.1438, -45.1)
  line L47 (-4.6187, -26.05) -> (9.3813, -26.05)
  line L48 (87.9625, -26.05) -> (87.9625, -12.05)
  line L49 (73.9625, -12.05) -> (73.9625, -26.05)
  line L50 (68.9125, -12.05) -> (54.9125, -12.05)
  line L51 (202.2625, -26.05) -> (202.2625, -12.05)
  line L52 (107.0125, -12.05) -> (93.0125, -12.05)
  line L53 (73.9625, -26.05) -> (87.9625, -26.05)
  line L54 (223.6938, -7) -> (223.6938, 7)
  line L55 (93.0125, -12.05) -> (93.0125, -26.05)
  line L56 (131.1125, -26.05) -> (145.1125, -26.05)
  line L57 (197.5, -7) -> (197.5, 7)
  line L58 (212.075, -26.05) -> (226.075, -26.05)
  line L59 (112.0625, -26.05) -> (126.0625, -26.05)
  line L60 (126.0625, -12.05) -> (112.0625, -12.05)
  line L61 (9.3813, -12.05) -> (-4.6187, -12.05)
  line L62 (212.075, -12.05) -> (212.075, -26.05)
  line L63 (145.1125, -26.05) -> (145.1125, -12.05)
  line L64 (35.8625, -12.05) -> (35.8625, -26.05)
  line L65 (150.1625, -26.05) -> (164.1625, -26.05)
  line L66 (209.6937, 7) -> (209.6937, -7)
  line L67 (49.8625, -12.05) -> (35.8625, -12.05)
  line L68 (87.9625, -12.05) -> (73.9625, -12.05)
  line L69 (183.2125, -12.05) -> (169.2125, -12.05)
  line L70 (223.6938, 7) -> (209.6937, 7)
  line L71 (183.5, 7) -> (183.5, -7)
  line L72 (126.0625, -26.05) -> (126.0625, -12.05)
  line L73 (169.2125, -26.05) -> (183.2125, -26.05)
  line L74 (54.9125, -12.05) -> (54.9125, -26.05)
  line L75 (64.4375, -31.1) -> (64.4375, -45.1)
  line L76 (140.35, -7) -> (140.35, 7)
  line L77 (16.8125, -12.05) -> (16.8125, -26.05)
  line L78 (140.6375, -31.1) -> (140.6375, -45.1)
  line L79 (159.4, -7) -> (159.4, 7)
  line L80 (209.6937, -7) -> (223.6938, -7)
  line L81 (14.1437, -45.1) -> (14.1437, -31.1)
  line L82 (226.075, -12.05) -> (212.075, -12.05)
  line L83 (59.3875, -31.1) -> (45.3875, -31.1)
  line L84 (45.3875, -45.1) -> (59.3875, -45.1)
  line L85 (45.1, 7) -> (31.1, 7)
  line L86 (188.2625, -26.05) -> (202.2625, -26.05)
  line L87 (107.0125, -26.05) -> (107.0125, -12.05)
  line L88 (68.9125, -26.05) -> (68.9125, -12.05)
  line L89 (150.1625, -12.05) -> (150.1625, -26.05)
  line L90 (112.0625, -12.05) -> (112.0625, -26.05)
  line L91 (164.1625, -12.05) -> (150.1625, -12.05)
  line L92 (-4.6187, -12.05) -> (-4.6187, -26.05)
  line L93 (9.3813, -26.05) -> (9.3813, -12.05)
  line L94 (16.8125, -26.05) -> (30.8125, -26.05)
  line L95 (30.8125, -12.05) -> (16.8125, -12.05)
  line L96 (49.8625, -26.05) -> (49.8625, -12.05)
  line L97 (188.2625, -12.05) -> (188.2625, -26.05)
  line L98 (169.2125, -12.05) -> (169.2125, -26.05)
  line L99 (30.8125, -26.05) -> (30.8125, -12.05)
  line L100 (35.8625, -26.05) -> (49.8625, -26.05)
  line L101 (183.2125, -26.05) -> (183.2125, -12.05)
  line L102 (97.4875, -45.1) -> (97.4875, -31.1)
  line L103 (26.3375, -45.1) -> (40.3375, -45.1)
  line L104 (192.7375, -31.1) -> (178.7375, -31.1)
  line L105 (116.5375, -45.1) -> (116.5375, -31.1)
  line L106 (50.15, -64.15) -> (64.15, -64.15)
  line L107 (26.3375, -31.1) -> (26.3375, -45.1)
  line L108 (-7, -50.15) -> (-7, -64.15)
  line L109 (135.5875, -31.1) -> (121.5875, -31.1)
  line L110 (159.6875, -31.1) -> (159.6875, -45.1)
  line L111 (140.6375, -45.1) -> (154.6375, -45.1)
  line L112 (12.05, -64.15) -> (26.05, -64.15)
  line L113 (211.7875, -31.1) -> (197.7875, -31.1)
  line L114 (40.3375, -31.1) -> (26.3375, -31.1)
  line L115 (78.4375, -45.1) -> (78.4375, -31.1)
  line L116 (7, -50.15) -> (-7, -50.15)
  line L117 (31.1, -50.15) -> (31.1, -64.15)
  line L118 (45.1, -50.15) -> (31.1, -50.15)
  line L119 (102.5375, -45.1) -> (116.5375, -45.1)
  line L120 (173.6875, -45.1) -> (173.6875, -31.1)
  line L121 (83.4875, -45.1) -> (97.4875, -45.1)
  line L122 (154.6375, -31.1) -> (140.6375, -31.1)
  line L123 (45.1, -64.15) -> (45.1, -50.15)
  line L124 (40.3375, -45.1) -> (40.3375, -31.1)
  line L125 (178.7375, -31.1) -> (178.7375, -45.1)
  line L126 (0.1438, -31.1) -> (0.1438, -45.1)
  line L127 (178.7375, -45.1) -> (192.7375, -45.1)
  line L128 (211.7875, -45.1) -> (211.7875, -31.1)
  line L129 (216.8375, -45.1) -> (230.8375, -45.1)
  line L130 (12.05, -50.15) -> (12.05, -64.15)
  line L131 (78.4375, -31.1) -> (64.4375, -31.1)
  line L132 (83.4875, -31.1) -> (83.4875, -45.1)
  line L133 (192.7375, -45.1) -> (192.7375, -31.1)
  line L134 (81.1062, -64.15) -> (95.1062, -64.15)
  line L135 (168.925, -50.15) -> (154.925, -50.15)
  line L136 (45.3875, -31.1) -> (45.3875, -45.1)
  line L137 (230.8375, -50.15) -> (216.8375, -50.15)
  line L138 (230.8375, -64.15) -> (230.8375, -50.15)
  line L139 (96.5443, -64.15) -> (103.5443, -64.15)
  line L140 (72.6683, -64.15) -> (79.6683, -64.15)
  line L141 (173.6875, -31.1) -> (159.6875, -31.1)
  line L142 (216.8375, -31.1) -> (216.8375, -45.1)
  line L143 (144.0255, -49.15) -> (137.0255, -49.15)
  line L144 (159.6875, -45.1) -> (173.6875, -45.1)
  line L145 (50.15, -50.15) -> (50.15, -64.15)
  line L146 (121.5875, -50.15) -> (121.5875, -64.15)
  line L147 (97.4875, -31.1) -> (83.4875, -31.1)
  line L148 (154.6375, -45.1) -> (154.6375, -31.1)
  line L149 (137.0255, -64.15) -> (144.0255, -64.15)
  line L150 (178.7375, -64.15) -> (192.7375, -64.15)
  line L151 (230.8375, -31.1) -> (216.8375, -31.1)
  line L152 (135.5875, -45.1) -> (135.5875, -31.1)
  line L153 (64.4375, -45.1) -> (78.4375, -45.1)
  line L154 (211.7875, -50.15) -> (197.7875, -50.15)
  line L155 (116.5375, -31.1) -> (102.5375, -31.1)
  line L156 (31.1, -64.15) -> (45.1, -64.15)
  line L157 (95.1062, -64.15) -> (95.1062, -50.15)
  line L158 (211.7875, -64.15) -> (211.7875, -50.15)
  line L159 (81.1062, -50.15) -> (81.1062, -64.15)
  line L160 (102.5375, -31.1) -> (102.5375, -45.1)
  line L161 (192.7375, -64.15) -> (192.7375, -50.15)
  line L162 (216.8375, -64.15) -> (230.8375, -64.15)
  line L163 (197.7875, -64.15) -> (211.7875, -64.15)
  line L164 (96.5443, -49.15) -> (96.5443, -64.15)
  line L165 (137.0255, -49.15) -> (137.0255, -64.15)
  line L166 (113.1495, -64.15) -> (120.1495, -64.15)
  line L167 (154.925, -50.15) -> (154.925, -64.15)
  line L168 (103.5442, -49.15) -> (96.5443, -49.15)
  line L169 (103.5442, -64.15) -> (103.5442, -49.15)
  line L170 (168.925, -64.15) -> (168.925, -50.15)
  line L171 (197.7875, -50.15) -> (197.7875, -64.15)
  line L172 (216.8375, -50.15) -> (216.8375, -64.15)
  line L173 (26.05, -64.15) -> (26.05, -50.15)
  line L174 (59.3875, -45.1) -> (59.3875, -31.1)
  line L175 (26.05, -50.15) -> (12.05, -50.15)
  line L176 (197.7875, -45.1) -> (211.7875, -45.1)
  line L177 (14.1437, -31.1) -> (0.1437, -31.1)
  line L178 (144.0255, -64.15) -> (144.0255, -49.15)
  line L179 (135.5875, -64.15) -> (135.5875, -50.15)
  line L180 (120.1495, -64.15) -> (120.1495, -49.15)
  line L181 (121.5875, -45.1) -> (135.5875, -45.1)
  line L182 (7, -64.15) -> (7, -50.15)
  line L183 (121.5875, -31.1) -> (121.5875, -45.1)
  line L184 (197.7875, -31.1) -> (197.7875, -45.1)
  line L185 (121.5875, -64.15) -> (135.5875, -64.15)
  line L186 (230.8375, -45.1) -> (230.8375, -31.1)
  line L187 (64.15, -50.15) -> (50.15, -50.15)
  line L188 (64.15, -64.15) -> (64.15, -50.15)
  line L189 (-7, -64.15) -> (7, -64.15)
  line L190 (120.1495, -49.15) -> (113.1495, -49.15)
  line L191 (72.6683, -49.15) -> (72.6683, -64.15)
  line L192 (113.1495, -49.15) -> (113.1495, -64.15)
  line L193 (135.5875, -50.15) -> (121.5875, -50.15)
  line L194 (192.7375, -50.15) -> (178.7375, -50.15)
  line L195 (79.6683, -64.15) -> (79.6683, -49.15)
  line L196 (95.1062, -50.15) -> (81.1062, -50.15)
  line L197 (178.7375, -50.15) -> (178.7375, -64.15)
  line L198 (79.6683, -49.15) -> (72.6683, -49.15)
  line L199 (154.925, -64.15) -> (168.925, -64.15)